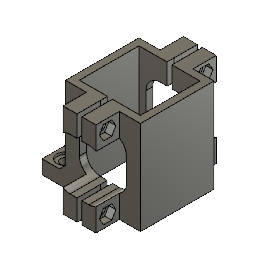
Brake Splitter Bracket v5 (Autodesk Fusion 360 design; units mm, degrees)
Autodesk Fusion 360 part; units mm, degrees
sketch "Sketch1" plane through (0, 0, 0) normal (0, 1, 0) x (1, 0, 0)
  line L0 (13, -12.7) -> (-13, -12.7)
  line L1 (-13, -12.7) -> (-13, 12.7)
  line L2 (-13, 12.7) -> (13, 12.7)
  line L3 (13, 12.7) -> (13, -12.7)
  line L4 (13, -12.7) -> (-13, 12.7) construction
  line L5 (-13, -12.7) -> (13, 12.7) construction
  line L6 (-16, -15.7) -> (-16, 15.7)
  line L7 (-7.0326, 15.7) -> (-7.0326, 25.7)
  line L8 (-7.0326, 25.7) -> (-1.0326, 25.7)
  line L9 (-1.0326, 25.7) -> (-1.0326, 15.7)
  line L10 (-16, 15.7) -> (-7.0326, 15.7)
  line L11 (0, -20) -> (0, 40) construction
  line L12 (-13, -12.7) -> (0, -12.7)
  line L13 (-13, -12.7) -> (-13, 12.7)
  line L14 (-13, 12.7) -> (-1.0896, 12.7)
  line L15 (-1.0326, 15.7) -> (-1.0896, 12.7)
  line L16 (-16, 15.7) -> (-26, 15.7)
  line L17 (-26, 15.7) -> (-26, 5.7)
  line L18 (-26, 5.7) -> (-16, 5.7)
  line L19 (-16, 5.7) -> (-16, 15.7)
  line L20 (-16, -15.7) -> (-26, -15.7)
  line L21 (-26, -15.7) -> (-26, -5.7)
  line L22 (-26, -5.7) -> (-16, -5.7)
  line L23 (-16, -5.7) -> (-16, -15.7)
  line L24 (20, 0) -> (-35, 0) construction
  line L25 (-7.0326, -15.7) -> (-7.0326, -25.7)
  line L26 (-7.0326, -25.7) -> (-1.0326, -25.7)
  line L27 (-1.0326, -25.7) -> (-1.0326, -15.7)
  line L28 (-1.0326, -15.7) -> (-1.0896, -12.7)
  line L29 (-16, -15.7) -> (-7.0326, -15.7)
  dimension "d1" = 26
  dimension "d2" = 25.4
  dimension "d4" = 6
  dimension "d29" = 10
  dimension "d30" = 10
  dimension "d31" = 10
  dimension "d32" = 10
  dimension "d45" = 3
  constraint horizontal L0
  constraint perpendicular L0 L1
  constraint parallel L0 L2
  constraint parallel L1 L3
  constraint coincident L4 origin
  constraint coincident L5 origin
  constraint vertical L7
  constraint horizontal L8
  constraint vertical L9
  constraint parallel L1 L6
  constraint midpoint L0 L12.end
  constraint perpendicular L11 L12
  constraint coincident L2 L14.end
  constraint perpendicular L11 L14
  constraint horizontal L29
  constraint horizontal L16
  constraint vertical L17
  constraint horizontal L18
  constraint vertical L19
  constraint horizontal L20
  constraint vertical L21
  constraint horizontal L22
  constraint vertical L23
  constraint horizontal L24
  constraint symmetric L9.end L24 L27.end
  constraint symmetric L7.start L24 L25.start
  constraint symmetric L7.end L24 L25.end
  constraint symmetric L8.end L24 L26.end
  constraint symmetric L14.end L24 L28.end
  measures "d1" distance of L1.end L2.end
  measures "d2" distance of L0.end L1.end
  measures "d4" distance of L9.end L7.start
  measures "d29" distance of L6.end L16.end
  measures "d30" distance of L6.end L18.end
  measures "d31" distance of L6.start L20.end
  measures "d32" distance of L6.start L22.end
  measures "d45" distance of L1 L6
extrude "Extrude1" add sketch "Sketch1" along normal blind 40 contours L0 L1 L2 L6 L7 L8 L9 L10 L12 L13 L14 L15 L19 L23 L25 L26 L27 L28 L29 makes body 1
sketch "Sketch2" plane through (0, 0, 15.7) normal (0, 0, 1) x (1, 0, 0)
  line L0 (-15.7, 0) -> (0, 0)
  line L1 (0, 0) -> (0, 40)
  line L2 (0, 40) -> (-15.7, 40)
  line L3 (-15.7, 40) -> (-15.7, 0)
  line L4 (-10, 9) -> (10, 9)
  line L5 (10, 9) -> (10, 31)
  line L6 (10, 31) -> (-10, 31)
  line L7 (-10, 31) -> (-10, 9)
  line L8 (-10, 9) -> (10, 31) construction
  line L9 (10, 9) -> (-10, 31) construction
  point P0 (0, 20)
  constraint horizontal L4
  constraint perpendicular L4 L5
  constraint parallel L4 L6
  constraint parallel L5 L7
  constraint coincident L8 P0
  constraint coincident L9 P0
  constraint midpoint L1 P0
extrude "Extrude3" add sketch "Sketch1" along normal blind 40 separate body contours L0 L1 L2 L3 L12 L13 L14 makes body 2
mirror "Mirror1" about plane through (0, 0, 0) normal (1, 0, 0) of "Extrude1" makes body 3
extrude "Extrude2" cut sketch "Sketch2" against normal through all from surface at 10 contours L1 L4 L6 L7 | L1 L4 L5 L6 bodies 1 3
hole "Hole1" at (-7.0326, 35.5, -20.7) direction (1, 0, 0) diameter 4.2 end through all counterbore diameter 7.2 counterbore depth 1.5 bodies 3 1
sketch "Sketch3" plane through (7.0326, 0, 0) normal (1, 0, 0) x (0, 0, -1)
  circle A0 centre (20.7, 35.5) radius 2.1
  line L0 (15.7, 31) -> (25.7, 31)
  line L1 (25.7, 31) -> (25.7, 40)
  line L2 (25.7, 40) -> (15.7, 40)
  line L3 (15.7, 40) -> (15.7, 31)
  line L4 (24.2, 35.5) -> (22.45, 38.5311)
  line L5 (22.45, 38.5311) -> (18.95, 38.5311)
  line L6 (18.95, 38.5311) -> (17.2, 35.5)
  line L7 (17.2, 35.5) -> (18.95, 32.4689)
  line L8 (18.95, 32.4689) -> (22.45, 32.4689)
  line L9 (22.45, 32.4689) -> (24.2, 35.5)
  point P0 (20.7, 35.5)
  dimension "d20" = 3.5
  constraint coincident P0 A0.centre
  measures "d20" distance of L4.start P0
extrude "Extrude4" cut sketch "Sketch3" against normal blind 3 contours L4 L5 L6 L7 L8 L9 bodies 3
ref_plane "WorkPlane1" through (8.5163, 20, 0) normal (0, 1, 0) x (0, 0, 1)
mirror "Mirror4" about plane through (0, 0, 0) normal (0, 0, 1) of "Hole1", "Extrude4"
mirror "Mirror2" about plane through (8.5163, 20, 0) normal (0, 1, 0) of "Hole1", "Extrude4", "Mirror4"
extrude "Extrude5" add sketch "Sketch1" along normal blind 6 contours L6 L20 L21 L22 L23 | L6 L16 L17 L18 L19 bodies 1
hole "Hole3" at (-21, 6, -10.7) direction (0, -1, 0) diameter 4.2 end through all counterbore diameter 7.2 counterbore depth 1 bodies 1
mirror "Mirror3" about plane through (0, 0, 0) normal (0, 0, 1) of "Hole3"
chamfer "Chamfer1" distance 2.5 angle 45 2 edges at (-16, 6, -10.7) (-16, 6, 10.7) on bodies 1
fillet "Fillet1" radius 6 4 edges at (-10, 9, -14.2) (-10, 31, -14.2) (10, 9, -14.2) (10, 31, -14.2) on bodies 1 3
fillet "Fillet1" radius 6 4 edges at (-10, 9, 14.2) (-10, 31, 14.2) (10, 9, 14.2) (10, 31, 14.2) on bodies 1 3
hidden bodies 2
